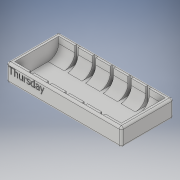
# Autodesk Inventor part: Thursday
Saved by Autodesk Inventor 2019.4 (Build 234330000, 330)
## iProperties
Created: 2020-10-20
Part Number: Thursday
Material: Generic
Document SubType Name: Modeling
Designer: daanswinters
Density: 1 g/cm^3
Appearance: Default
Author: daanswinters
Autodesk Inventor part; units mm, degrees
ref_plane "YZ Plane" through (0, 0, 0) normal (1, 0, 0) x (0, 1, 0)
ref_plane "XZ Plane" through (0, 0, 0) normal (0, 1, 0) x (-1, 0, 0)
ref_plane "XY Plane" through (0, 0, 0) normal (0, 0, 1) x (1, 0, 0)
sketch "Sketch1" plane through (0, 0, 0) normal (0, 0, 1) x (1, 0, 0)
  line L0 (55, -8.5) -> (-55, -8.5)
  line L1 (-55, -8.5) -> (-55, 8.5)
  line L2 (-55, 8.5) -> (55, 8.5)
  line L3 (55, 8.5) -> (55, -8.5)
  line L4 (55, -8.5) -> (-55, 8.5) construction
  line L5 (-55, -8.5) -> (55, 8.5) construction
  point P0 (0, 0)
  dimension "d0" = 110
  dimension "d1" = 17
  constraints: 12 end point, 2 midpoint, 2 parallel, 1 horizontal, 1 perpendicular
  measures "d0" distance of L1.end L2.end
  measures "d1" distance of L0.end L1.end
extrude "Extrusion1" add sketch "Sketch1" along normal blind 50
sketch "Sketch2" plane through (-55, 8.5, 0) normal (0, 1, 0) x (1, 0, 0)
  line L0 (0, 0) -> (0, -50) projected
  line L1 (110, -50) -> (0, -50)
  line L2 (0, -50) -> (0, 0)
  line L3 (0, 0) -> (110, 0)
  line L4 (110, 0) -> (110, -50)
  line L5 (110, -50) -> (0, 0) construction
  line L6 (0, -50) -> (110, 0) construction
  line L7 (106, -46) -> (106, -4)
  line L8 (4, -4) -> (4, -46)
  line L9 (56.15, -2) -> (53.85, -2)
  line L10 (53.85, -48) -> (56.15, -48)
  line L11 (56.15, -2) -> (53.85, -48) construction
  line L12 (53.85, -2) -> (56.15, -48) construction
  line L13 (73.15, -2) -> (70.85, -2)
  line L14 (70.85, -48) -> (73.15, -48)
  line L15 (73.15, -2) -> (70.85, -48) construction
  line L16 (70.85, -2) -> (73.15, -48) construction
  line L17 (0, -25) -> (110, -25) construction
  line L18 (87.85, -2) -> (90.15, -2)
  line L19 (90.15, -48) -> (87.85, -48)
  line L20 (87.85, -2) -> (90.15, -48) construction
  line L21 (90.15, -2) -> (87.85, -48) construction
  line L22 (36.85, -2) -> (39.15, -2)
  line L23 (39.15, -48) -> (36.85, -48)
  line L24 (36.85, -2) -> (39.15, -48) construction
  line L25 (39.15, -2) -> (36.85, -48) construction
  line L26 (19.85, -2) -> (22.15, -2)
  line L27 (22.15, -48) -> (19.85, -48)
  line L28 (19.85, -2) -> (22.15, -48) construction
  line L29 (22.15, -2) -> (19.85, -48) construction
  line L30 (90.15, -2) -> (90.15, -4)
  line L31 (90.15, -46) -> (90.15, -48)
  line L32 (87.85, -48) -> (87.85, -46)
  line L33 (87.85, -4) -> (87.85, -2)
  line L34 (73.15, -48) -> (73.15, -46)
  line L35 (73.15, -4) -> (73.15, -2)
  line L36 (70.85, -2) -> (70.85, -4)
  line L37 (70.85, -46) -> (70.85, -48)
  line L38 (56.15, -4) -> (56.15, -2)
  line L39 (53.85, -2) -> (53.85, -4)
  line L40 (53.85, -46) -> (53.85, -48)
  line L41 (56.15, -48) -> (56.15, -46)
  line L42 (39.15, -2) -> (39.15, -4)
  line L43 (39.15, -46) -> (39.15, -48)
  line L44 (36.85, -48) -> (36.85, -46)
  line L45 (36.85, -4) -> (36.85, -2)
  line L46 (22.15, -2) -> (22.15, -4)
  line L47 (19.85, -48) -> (19.85, -46)
  line L48 (19.85, -4) -> (19.85, -2)
  line L49 (22.15, -46) -> (22.15, -48)
  line L50 (4, -46) -> (19.95, -46)
  line L51 (22.05, -46) -> (36.95, -46)
  line L52 (39.05, -46) -> (53.95, -46)
  line L53 (56.05, -46) -> (70.95, -46)
  line L54 (73.05, -46) -> (87.95, -46)
  line L55 (90.05, -46) -> (106, -46)
  line L56 (106, -4) -> (90.05, -4)
  line L57 (87.95, -4) -> (73.05, -4)
  line L58 (70.95, -4) -> (56.05, -4)
  line L59 (53.95, -4) -> (39.05, -4)
  line L60 (36.95, -4) -> (22.05, -4)
  line L61 (19.95, -4) -> (4, -4)
  point P0 (55, 0)
  point P1 (55, -25)
  point P2 (72, -25)
  point P3 (89, -25)
  point P4 (38, -25)
  point P5 (21, -25)
  dimension "d4" = 65.556
  dimension "d5" = 110
  dimension "d7" = 2.3
  dimension "d8" = 46
  dimension "d9" = 2.3
  dimension "d10" = 46
  dimension "d11" = 0
  dimension "d12" = 2.3
  dimension "d13" = 46
  dimension "d14" = 2.3
  dimension "d15" = 46
  dimension "d16" = 2.3
  dimension "d17" = 46
  dimension "d18" = 17
  dimension "d19" = 17
  dimension "d20" = 17
  dimension "d21" = 17
  dimension "d22" = 2.862
  dimension "d23" = 2.862
  dimension "d24" = 106
  dimension "d25" = 4
  dimension "d26" = 42
  dimension "d27" = 2
  dimension "d28" = 0
  dimension "d29" = 42
  dimension "d30" = 0
  dimension "d31" = 42
  dimension "d32" = 0
  dimension "d33" = 42
  dimension "d34" = 0
  dimension "d35" = 42
  dimension "d36" = 0
  dimension "d37" = 42
  constraints: 122 end point, 73 parallel, 43 point on line, 17 perpendicular, 14 midpoint, 6 horizontal
  measures "d4" angle of L5 L0
  measures "d5" distance between parallel lines of L4 L0
  measures "d7" distance of L10.end L10.start
  measures "d8" distance of L10.start L9.end
  measures "d9" distance of L14.end L14.start
  measures "d10" distance of L14.start L13.end
  measures "d11" distance from line of L17 point (72, -25)
  measures "d12" distance of L19.start L19.end
  measures "d13" distance of L18.end L19.start
  measures "d14" distance of L23.start L23.end
  measures "d15" distance of L22.end L23.start
  measures "d16" distance of L27.start L27.end
  measures "d17" distance of L26.end L27.start
  measures "d18" distance of point (72, -25) point (55, -25)
  measures "d19" distance of point (89, -25) point (72, -25)
  measures "d20" distance of point (38, -25) point (55, -25)
  measures "d21" distance of point (21, -25) point (38, -25)
  measures "d22" angle of L0 L20
  measures "d23" angle of L0 L21
  measures "d24" distance between parallel lines of L7 L0
  measures "d25" distance between parallel lines of L8 L0
  measures "d26" distance between parallel lines of L56 L55
  measures "d27" distance between parallel lines of L56 L18
  measures "d28" distance between parallel lines of L56 L57
  measures "d29" distance between parallel lines of L56 L54
  measures "d30" distance between parallel lines of L56 L58
  measures "d31" distance between parallel lines of L56 L53
  measures "d32" distance between parallel lines of L56 L59
  measures "d33" distance between parallel lines of L56 L52
  measures "d34" distance between parallel lines of L56 L60
  measures "d35" distance between parallel lines of L56 L51
  measures "d36" distance between parallel lines of L56 L61
  measures "d37" distance between parallel lines of L56 L50
extrude "Extrusion2" cut sketch "Sketch2" against normal blind 16 contours L55 L31 L19 L32 L54 L34 L14 L37 L53 L41 L10 L40 L52 L43 L23 L44 L51 L49 L27 L47 L50 L8 L61 L48 L26 L46 L60 L45 L22 L42 L59 L39 L9 L38 L58 L36 L13 L35 L57 L33 L18 L30 L56 L7
fillet "Fillet1" radius 2 12 edges at (-55, 0, 50) (-55, 0, 0) (55, 0, 50) (55, 0, 0) (0, 8.5, 50) (-55, 8.5, 25) (0, 8.5, 0) (55, 8.5, 25) (55, -8.5, 25) (0, -8.5, 50) (-55, -8.5, 25) (0, -8.5, 0)
fillet "Fillet2" radius 10 6 edges at (-43.075, -7.5, 4) (-25.5, -7.5, 4) (-8.5, -7.5, 4) (8.5, -7.5, 4) (25.5, -7.5, 4) (43.075, -7.5, 4)
sketch "Sketch3" plane through (35.15, 8.5, 4) normal (0, 1, 0) x (1, 0, 0)
  line L0 (-70.3, -44) -> (-70.3, -42) projected
  line L1 (-51, 2) -> (-53.3, 2)
  line L2 (-34, 2) -> (-34, 0) projected
  line L3 (-36.3, -44) -> (-36.3, -42) projected
  line L4 (-19.3, -44) -> (-19.3, -42) projected
  line L5 (-2.3, -44) -> (-2.3, -42) projected
  line L6 (0, 2) -> (0, 0) projected
  line L7 (-19.8, 2) -> (-16.5, 2)
  line L8 (-16.5, 2) -> (-16.5, -44)
  line L9 (-16.5, -44) -> (-19.8, -44)
  line L10 (-19.8, -44) -> (-19.8, 2)
  line L11 (-19.8, 2) -> (-16.5, -44) construction
  line L12 (-16.5, 2) -> (-19.8, -44) construction
  line L13 (-2.8, -44) -> (0.5, -44)
  line L14 (0.5, -44) -> (0.5, 2)
  line L15 (0.5, 2) -> (-2.8, 2)
  line L16 (-2.8, 2) -> (-2.8, -44)
  line L17 (-2.8, -44) -> (0.5, 2) construction
  line L18 (0.5, -44) -> (-2.8, 2) construction
  line L19 (-36.8, -44) -> (-33.5, -44)
  line L20 (-33.5, -44) -> (-33.5, 2)
  line L21 (-33.5, 2) -> (-36.8, 2)
  line L22 (-36.8, 2) -> (-36.8, -44)
  line L23 (-36.8, -44) -> (-33.5, 2) construction
  line L24 (-33.5, -44) -> (-36.8, 2) construction
  line L25 (-51, 2) -> (-36.3, 2) projected
  line L26 (-53.8, -44) -> (-50.5, -44)
  line L27 (-50.5, -44) -> (-50.5, 2)
  line L28 (-50.5, 2) -> (-53.8, 2)
  line L29 (-53.8, 2) -> (-53.8, -44)
  line L30 (-53.8, -44) -> (-50.5, 2) construction
  line L31 (-50.5, -44) -> (-53.8, 2) construction
  line L32 (-53.3, -44) -> (-68, -44) projected
  line L33 (-70.8, 2) -> (-67.5, 2)
  line L34 (-67.5, 2) -> (-67.5, -44)
  line L35 (-67.5, -44) -> (-70.8, -44)
  line L36 (-70.8, -44) -> (-70.8, 2)
  line L37 (-70.8, 2) -> (-67.5, -44) construction
  line L38 (-67.5, 2) -> (-70.8, -44) construction
  point P0 (-35.15, 4)
  point P1 (-68, 2)
  point P2 (-17, 2)
  point P3 (-18.15, -21)
  point P4 (-1.15, -21)
  point P5 (-35.15, -21)
  point P6 (-52.15, -21)
  point P7 (-69.15, -21)
  dimension "d42" = 3.3
  dimension "d43" = 46
  dimension "d44" = 3.3
  dimension "d45" = 3.3
  dimension "d46" = 3.3
  dimension "d47" = 3.3
  dimension "d48" = 90
  dimension "d49" = 0.5
  dimension "d50" = 16.5
  dimension "d51" = 33.5
  dimension "d52" = 50.5
  dimension "d53" = 67.5
  dimension "d54" = 46
  dimension "d55" = 0
  dimension "d56" = 53.3
  constraints: 62 end point, 14 parallel, 10 midpoint, 5 horizontal, 5 perpendicular, 3 point on line
  measures "d42" distance of L8.end L9.end
  measures "d43" distance of L7.end L8.end
  measures "d44" distance of L15.end L14.end
  measures "d45" distance of L21.end L20.end
  measures "d46" distance of L28.end L27.end
  measures "d47" distance of L34.end L35.end
  measures "d48" angle of L6 L1
  measures "d49" distance between parallel lines of L6 L14
  measures "d50" distance between parallel lines of L6 L8
  measures "d51" distance between parallel lines of L6 L20
  measures "d52" distance between parallel lines of L6 L27
  measures "d53" distance between parallel lines of L6 L34
  measures "d54" distance between parallel lines of L25 L9
  measures "d55" distance between parallel lines of L15 L25
  measures "d56" distance from line of L1.end L6
extrude "Extrusion3" cut sketch "Sketch3" against normal blind 16
sketch "Sketch4" plane through (0, 0, 50) normal (0, 0, 1) x (1, 0, 0)
  line L0 (-52.9749, 6.5012) -> (53.0345, 6.5012) construction
  line L1 (53.0345, 6.5012) -> (53.0345, -6.5247) construction
  line L2 (53.0345, -6.5247) -> (-52.9749, -6.5247) construction
  line L3 (-52.9749, -6.5247) -> (-52.9749, 6.5012) construction
  line L4 (-50.9334, 0.1294) -> (-50.9334, 5.5077)
  line L5 (-50.9334, 5.5077) -> (-52.9799, 5.5077)
  line L6 (-52.9799, 5.5077) -> (-52.9799, 6.2294)
  line L7 (-52.9799, 6.2294) -> (-48.0761, 6.2294)
  line L8 (-48.0761, 6.2294) -> (-48.0761, 5.5077)
  line L9 (-48.0761, 5.5077) -> (-50.1227, 5.5077)
  line L10 (-50.1227, 5.5077) -> (-50.1227, 0.1294)
  line L11 (-50.1227, 0.1294) -> (-50.9334, 0.1294)
  line L12 (-43.9238, 0.1294) -> (-44.6949, 0.1294)
  line L13 (-44.6949, 0.1294) -> (-44.6949, 2.7394)
  spline S0 degree 2 poles (-44.6949, 2.7394) (-44.6949, 3.0558) (-44.7543, 3.5995) (-44.8432, 3.7627) knots 0 0 0 1 2 2 2
  spline S1 degree 2 poles (-44.8432, 3.7627) (-44.9372, 3.9357) (-45.2733, 4.1038) (-45.56, 4.1038) knots 0 0 0 1 2 2 2
  spline S2 degree 2 poles (-45.56, 4.1038) (-45.8467, 4.1038) (-46.4547, 3.7973) (-46.7464, 3.5501) knots 0 0 0 1 2 2 2
  line L14 (-46.7464, 3.5501) -> (-46.7464, 0.1294)
  line L15 (-46.7464, 0.1294) -> (-47.5176, 0.1294)
  line L16 (-47.5176, 0.1294) -> (-47.5176, 6.5012)
  line L17 (-47.5176, 6.5012) -> (-46.7464, 6.5012)
  line L18 (-46.7464, 6.5012) -> (-46.7464, 4.1977)
  spline S3 degree 2 poles (-46.7464, 4.1977) (-46.4004, 4.5091) (-45.733, 4.8354) (-45.3573, 4.8354) knots 0 0 0 1 2 2 2
  spline S4 degree 2 poles (-45.3573, 4.8354) (-44.6851, 4.8354) (-43.9238, 3.9456) (-43.9238, 3.1003) knots 0 0 0 1 2 2 2
  line L19 (-43.9238, 3.1003) -> (-43.9238, 0.1294)
  line L20 (-39.2821, 0.1294) -> (-40.0532, 0.1294)
  line L21 (-40.0532, 0.1294) -> (-40.0532, 0.6336)
  spline S5 degree 2 poles (-40.0532, 0.6336) (-40.4091, 0.3222) (-41.0468, 0.0008) (-41.4423, 0.0008) knots 0 0 0 1 2 2 2
  spline S6 degree 2 poles (-41.4423, 0.0008) (-41.7389, 0.0008) (-42.2678, 0.1986) (-42.4606, 0.4111) knots 0 0 0 1 2 2 2
  spline S7 degree 2 poles (-42.4606, 0.4111) (-42.6583, 0.6237) (-42.8758, 1.2713) (-42.8758, 1.7359) knots 0 0 0 1 2 2 2
  line L22 (-42.8758, 1.7359) -> (-42.8758, 4.7068)
  line L23 (-42.8758, 4.7068) -> (-42.1047, 4.7068)
  line L24 (-42.1047, 4.7068) -> (-42.1047, 2.0968)
  spline S8 degree 2 poles (-42.1047, 2.0968) (-42.1047, 1.731) (-42.0503, 1.2515) (-41.9564, 1.0735) knots 0 0 0 1 2 2 2
  spline S9 degree 2 poles (-41.9564, 1.0735) (-41.8624, 0.8956) (-41.5411, 0.7324) (-41.2396, 0.7324) knots 0 0 0 1 2 2 2
  spline S10 degree 2 poles (-41.2396, 0.7324) (-40.9578, 0.7324) (-40.3201, 1.0538) (-40.0532, 1.2861) knots 0 0 0 1 2 2 2
  line L25 (-40.0532, 1.2861) -> (-40.0532, 4.7068)
  line L26 (-40.0532, 4.7068) -> (-39.2821, 4.7068)
  line L27 (-39.2821, 4.7068) -> (-39.2821, 0.1294)
  line L28 (-35.7377, 3.8813) -> (-35.7773, 3.8813)
  spline S11 degree 2 poles (-35.7773, 3.8813) (-35.8663, 3.906) (-36.059, 3.9159) (-36.1925, 3.9159) knots 0 0 0 1 2 2 2
  spline S12 degree 2 poles (-36.1925, 3.9159) (-36.5039, 3.9159) (-37.1169, 3.644) (-37.3937, 3.3771) knots 0 0 0 1 2 2 2
  line L29 (-37.3937, 3.3771) -> (-37.3937, 0.1294)
  line L30 (-37.3937, 0.1294) -> (-38.1649, 0.1294)
  line L31 (-38.1649, 0.1294) -> (-38.1649, 4.7068)
  line L32 (-38.1649, 4.7068) -> (-37.3937, 4.7068)
  line L33 (-37.3937, 4.7068) -> (-37.3937, 4.0247)
  spline S13 degree 2 poles (-37.3937, 4.0247) (-36.9735, 4.4004) (-36.3458, 4.7068) (-36.0492, 4.7068) knots 0 0 0 1 2 2 2
  spline S14 degree 2 poles (-36.0492, 4.7068) (-35.9305, 4.7068) (-35.8119, 4.697) (-35.7377, 4.6821) knots 0 0 0 1 2 2 2
  line L34 (-35.7377, 4.6821) -> (-35.7377, 3.8813)
  spline S15 degree 2 poles (-33.9038, 0.0206) (-34.3635, 0.0206) (-35.1594, 0.2678) (-35.4214, 0.4062) knots 0 0 0 1 2 2 2
  line L35 (-35.4214, 0.4062) -> (-35.4214, 1.2713)
  line L36 (-35.4214, 1.2713) -> (-35.3818, 1.2713)
  spline S16 degree 2 poles (-35.3818, 1.2713) (-35.2829, 1.1922) (-35.016, 1.0043) (-34.7936, 0.9005) knots 0 0 0 1 2 2 2
  spline S17 degree 2 poles (-34.7936, 0.9005) (-34.6008, 0.8066) (-34.1262, 0.6682) (-33.8741, 0.6682) knots 0 0 0 1 2 2 2
  spline S18 degree 2 poles (-33.8741, 0.6682) (-33.6912, 0.6682) (-33.271, 0.7522) (-33.1722, 0.8214) knots 0 0 0 1 2 2 2
  spline S19 degree 2 poles (-33.1722, 0.8214) (-33.0288, 0.9153) (-32.9003, 1.1279) (-32.9003, 1.3454) knots 0 0 0 1 2 2 2
  spline S20 degree 2 poles (-32.9003, 1.3454) (-32.9003, 1.6173) (-33.1969, 1.8991) (-33.5775, 1.993) knots 0 0 0 1 2 2 2
  spline S21 degree 2 poles (-33.5775, 1.993) (-33.7258, 2.0276) (-34.2004, 2.1265) (-34.403, 2.1808) knots 0 0 0 1 2 2 2
  spline S22 degree 2 poles (-34.403, 2.1808) (-34.927, 2.3341) (-35.4016, 2.9668) (-35.4016, 3.4166) knots 0 0 0 1 2 2 2
  spline S23 degree 2 poles (-35.4016, 3.4166) (-35.4016, 4.0395) (-34.4673, 4.8156) (-33.6962, 4.8156) knots 0 0 0 1 2 2 2
  spline S24 degree 2 poles (-33.6962, 4.8156) (-33.3155, 4.8156) (-32.5444, 4.6277) (-32.2824, 4.4844) knots 0 0 0 1 2 2 2
  line L37 (-32.2824, 4.4844) -> (-32.2824, 3.6589)
  line L38 (-32.2824, 3.6589) -> (-32.3219, 3.6589)
  spline S25 degree 2 poles (-32.3219, 3.6589) (-32.6185, 3.8961) (-33.3402, 4.168) (-33.711, 4.168) knots 0 0 0 1 2 2 2
  spline S26 degree 2 poles (-33.711, 4.168) (-34.0916, 4.168) (-34.6156, 3.8467) (-34.6156, 3.5254) knots 0 0 0 1 2 2 2
  spline S27 degree 2 poles (-34.6156, 3.5254) (-34.6156, 3.2337) (-34.3042, 2.952) (-33.9582, 2.863) knots 0 0 0 1 2 2 2
  spline S28 degree 2 poles (-33.9582, 2.863) (-33.7901, 2.8185) (-33.365, 2.7295) (-33.1326, 2.6752) knots 0 0 0 1 2 2 2
  spline S29 degree 2 poles (-33.1326, 2.6752) (-32.6284, 2.5466) (-32.1143, 1.9584) (-32.1143, 1.4492) knots 0 0 0 1 2 2 2
  spline S30 degree 2 poles (-32.1143, 1.4492) (-32.1143, 1.1526) (-32.3466, 0.6286) (-32.574, 0.4359) knots 0 0 0 1 2 2 2
  spline S31 degree 2 poles (-32.574, 0.4359) (-32.8163, 0.2332) (-33.4342, 0.0206) (-33.9038, 0.0206) knots 0 0 0 1 2 2 2
  line L39 (-27.8779, 0.1294) -> (-28.6491, 0.1294)
  line L40 (-28.6491, 0.1294) -> (-28.6491, 0.594)
  spline S32 degree 2 poles (-28.6491, 0.594) (-28.827, 0.4457) (-29.089, 0.248) (-29.267, 0.164) knots 0 0 0 1 2 2 2
  spline S33 degree 2 poles (-29.267, 0.164) (-29.4301, 0.0849) (-29.7811, 0.0008) (-30.0134, 0.0008) knots 0 0 0 1 2 2 2
  spline S34 degree 2 poles (-30.0134, 0.0008) (-30.3891, 0.0008) (-31.0218, 0.3123) (-31.2443, 0.6138) knots 0 0 0 1 2 2 2
  spline S35 degree 2 poles (-31.2443, 0.6138) (-31.4667, 0.9153) (-31.7139, 1.8051) (-31.7139, 2.3835) knots 0 0 0 1 2 2 2
  spline S36 degree 2 poles (-31.7139, 2.3835) (-31.7139, 2.9866) (-31.4025, 3.8665) (-31.1306, 4.1977) knots 0 0 0 1 2 2 2
  spline S37 degree 2 poles (-31.1306, 4.1977) (-30.8785, 4.4943) (-30.1716, 4.8354) (-29.7811, 4.8354) knots 0 0 0 1 2 2 2
  spline S38 degree 2 poles (-29.7811, 4.8354) (-29.44, 4.8354) (-28.9308, 4.6821) (-28.6491, 4.5239) knots 0 0 0 1 2 2 2
  line L41 (-28.6491, 4.5239) -> (-28.6491, 6.5012)
  line L42 (-28.6491, 6.5012) -> (-27.8779, 6.5012)
  line L43 (-27.8779, 6.5012) -> (-27.8779, 0.1294)
  line L44 (-28.6491, 1.2416) -> (-28.6491, 3.8863)
  spline S39 degree 2 poles (-28.6491, 3.8863) (-28.9358, 4.0247) (-29.3906, 4.1285) (-29.6526, 4.1285) knots 0 0 0 1 2 2 2
  spline S40 degree 2 poles (-29.6526, 4.1285) (-30.2458, 4.1285) (-30.918, 3.2387) (-30.918, 2.3983) knots 0 0 0 1 2 2 2
  spline S41 degree 2 poles (-30.918, 2.3983) (-30.918, 1.5876) (-30.4039, 0.7324) (-29.8355, 0.7324) knots 0 0 0 1 2 2 2
  spline S42 degree 2 poles (-29.8355, 0.7324) (-29.5339, 0.7324) (-28.921, 1.0093) (-28.6491, 1.2416) knots 0 0 0 1 2 2 2
  spline S43 degree 2 poles (-24.21, 0.6138) (-24.3039, 0.5446) (-24.6203, 0.2974) (-24.7686, 0.2233) knots 0 0 0 1 2 2 2
  spline S44 degree 2 poles (-24.7686, 0.2233) (-24.9713, 0.1145) (-25.3519, 0.0008) (-25.6979, 0.0008) knots 0 0 0 1 2 2 2
  spline S45 degree 2 poles (-25.6979, 0.0008) (-25.9797, 0.0008) (-26.4889, 0.2134) (-26.6817, 0.4062) knots 0 0 0 1 2 2 2
  spline S46 degree 2 poles (-26.6817, 0.4062) (-26.8646, 0.594) (-27.087, 1.1477) (-27.087, 1.4542) knots 0 0 0 1 2 2 2
  spline S47 degree 2 poles (-27.087, 1.4542) (-27.087, 1.9287) (-26.6866, 2.601) (-26.2516, 2.7938) knots 0 0 0 1 2 2 2
  spline S48 degree 2 poles (-26.2516, 2.7938) (-25.866, 2.9718) (-24.818, 3.1052) (-24.21, 3.1398) knots 0 0 0 1 2 2 2
  line L45 (-24.21, 3.1398) -> (-24.21, 3.2881)
  spline S49 degree 2 poles (-24.21, 3.2881) (-24.21, 3.5551) (-24.3731, 3.8863) (-24.5214, 3.9802) knots 0 0 0 1 2 2 2
  spline S50 degree 2 poles (-24.5214, 3.9802) (-24.6697, 4.0741) (-25.0949, 4.1334) (-25.3223, 4.1334) knots 0 0 0 1 2 2 2
  spline S51 degree 2 poles (-25.3223, 4.1334) (-25.5892, 4.1334) (-26.3109, 3.9752) (-26.6718, 3.822) knots 0 0 0 1 2 2 2
  line L46 (-26.6718, 3.822) -> (-26.7163, 3.822)
  line L47 (-26.7163, 3.822) -> (-26.7163, 4.608)
  spline S52 degree 2 poles (-26.7163, 4.608) (-26.5037, 4.6673) (-25.7078, 4.8156) (-25.3173, 4.8156) knots 0 0 0 1 2 2 2
  spline S53 degree 2 poles (-25.3173, 4.8156) (-24.8428, 4.8156) (-24.1952, 4.6673) (-23.9381, 4.4745) knots 0 0 0 1 2 2 2
  spline S54 degree 2 poles (-23.9381, 4.4745) (-23.686, 4.2867) (-23.4389, 3.6885) (-23.4389, 3.2585) knots 0 0 0 1 2 2 2
  line L48 (-23.4389, 3.2585) -> (-23.4389, 0.1294)
  line L49 (-23.4389, 0.1294) -> (-24.21, 0.1294)
  line L50 (-24.21, 0.1294) -> (-24.21, 0.6138)
  line L51 (-24.21, 1.2564) -> (-24.21, 2.5269)
  spline S55 degree 2 poles (-24.21, 2.5269) (-24.4868, 2.5021) (-25.3223, 2.4181) (-25.5842, 2.339) knots 0 0 0 1 2 2 2
  spline S56 degree 2 poles (-25.5842, 2.339) (-25.8907, 2.2451) (-26.2911, 1.8546) (-26.2911, 1.5085) knots 0 0 0 1 2 2 2
  spline S57 degree 2 poles (-26.2911, 1.5085) (-26.2911, 1.1131) (-25.8462, 0.7127) (-25.4211, 0.7127) knots 0 0 0 1 2 2 2
  spline S58 degree 2 poles (-25.4211, 0.7127) (-25.0603, 0.7127) (-24.4671, 1.0241) (-24.21, 1.2564) knots 0 0 0 1 2 2 2
  line L52 (-18.7625, 4.7068) -> (-21.2243, -1.5563)
  line L53 (-21.2243, -1.5563) -> (-22.0498, -1.5563)
  line L54 (-22.0498, -1.5563) -> (-21.2292, 0.3518)
  line L55 (-21.2292, 0.3518) -> (-22.8902, 4.7068)
  line L56 (-22.8902, 4.7068) -> (-22.0597, 4.7068)
  line L57 (-22.0597, 4.7068) -> (-20.809, 1.3158)
  line L58 (-20.809, 1.3158) -> (-19.5633, 4.7068)
  line L59 (-19.5633, 4.7068) -> (-18.7625, 4.7068)
  point P0 (0, 0)
  constraints: 2 other
extrude "Extrusion4" cut sketch "Sketch4" against normal blind 0.5
fillet "Fillet3" radius 10 6 edges at (-43.325, -7.5, 46) (-25.5, -7.5, 46) (-8.5, -7.5, 46) (8.5, -7.5, 46) (25.5, -7.5, 46) (43.325, -7.5, 46)
body "Solid1"
